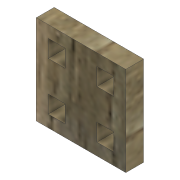
# Autodesk Inventor part: motor_middle
Saved by Autodesk Inventor 2020 (Build 240168000, 168)
## iProperties
Created: 2021-05-10
Part Number: motor_middle
Material: Generic
Document SubType Name: Modeling
Designer: Hsu Daniel
Density: 1 g/cm^3
Appearance: Driftwood
Author: Hsu Daniel
Autodesk Inventor part; units mm, degrees
ref_plane "YZ Plane" through (0, 0, 0) normal (1, 0, 0) x (0, 1, 0)
ref_plane "XZ Plane" through (0, 0, 0) normal (0, 1, 0) x (-1, 0, 0)
ref_plane "XY Plane" through (0, 0, 0) normal (0, 0, 1) x (1, 0, 0)
sketch "Sketch1" plane through (0, 0, 0) normal (0, 0, 1) x (1, 0, 0)
  line L0 (-2, -1.5) -> (2, -1.5)
  line L1 (2, 1.5) -> (-2, 1.5)
  arc A0 (-2, 1.5) -> (-2, -1.5) centre (0, 0) ccw
  arc A1 (2, -1.5) -> (2, 1.5) centre (0, 0) ccw
  line L2 (-7.5, -7.5) -> (7.5, -7.5)
  line L3 (7.5, -7.5) -> (7.5, 7.5)
  line L4 (7.5, 7.5) -> (-7.5, 7.5)
  line L5 (-7.5, 7.5) -> (-7.5, -7.5)
  line L6 (-7.5, -7.5) -> (7.5, 7.5) construction
  line L7 (7.5, -7.5) -> (-7.5, 7.5) construction
  line L8 (-5.5, 2.58) -> (-2.66, 2.58)
  line L9 (-2.66, 2.58) -> (-2.66, 5.5)
  line L10 (-2.66, 5.5) -> (-5.5, 5.5)
  line L11 (-5.5, 5.5) -> (-5.5, 2.58)
  line L12 (0, 0) -> (0, 4.08) construction
  line L13 (0, 0) -> (5.4269, 0) construction
  line L14 (2.66, 2.58) -> (2.66, 5.5)
  line L15 (2.66, 5.5) -> (5.5, 5.5)
  line L16 (5.5, 5.5) -> (5.5, 2.58)
  line L17 (5.5, 2.58) -> (2.66, 2.58)
  line L18 (2.66, -2.58) -> (2.66, -5.5)
  line L19 (5.5, -2.58) -> (2.66, -2.58)
  line L20 (5.5, -5.5) -> (5.5, -2.58)
  line L21 (2.66, -5.5) -> (5.5, -5.5)
  line L22 (-5.5, -2.58) -> (-2.66, -2.58)
  line L23 (-2.66, -5.5) -> (-5.5, -5.5)
  line L24 (-5.5, -5.5) -> (-5.5, -2.58)
  line L25 (-2.66, -2.58) -> (-2.66, -5.5)
  point P0 (0, 0)
  point P1 (0, -4.08)
  point P2 (0, 0)
  dimension "d0" = 4
  dimension "d1" = 2.5
  dimension "d2" = 15
  dimension "d4" = 2.84
  dimension "d5" = 2.92
  dimension "d6" = 2
  dimension "d7" = 2
  constraints: 52 end point, 13 symmetric about line, 5 parallel, 4 horizontal, 4 point on circle, 3 midpoint, 2 centre point, 2 coincident, 2 equal length, 2 perpendicular, 1 concentric, 1 vertical
  measures "d0" distance of L1.start L1.end
  measures "d1" radius of A1
  measures "d2" distance of L4.end L4.start
  measures "d4" distance of L10.end L9.end
  measures "d5" distance of L9.start L9.end
  measures "d6" distance between parallel lines of L4 L10
  measures "d7" distance between parallel lines of L5 L11
extrude "Extrusion1" add sketch "Sketch1" along normal blind 3 contours A0 L1 A1 L0 | L5 L4 L3 L2
body "Solid1"
